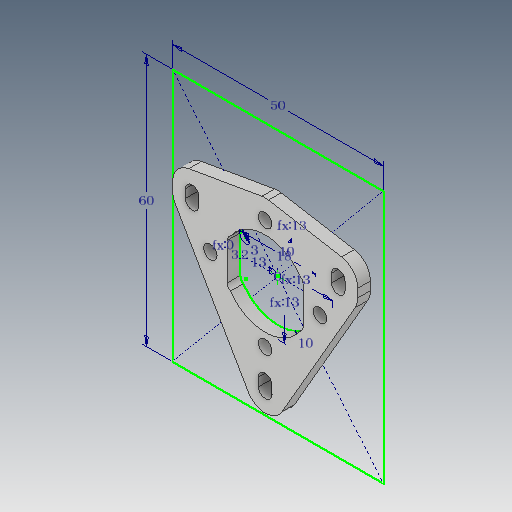
# Autodesk Inventor part: RS555-71Mount
Saved by Autodesk Inventor 2019.4 (Build 234330000, 330)
## iProperties
Created: 2019-06-16
Part Number: RS555-71Mount
Material: Generic
Document SubType Name: Modeling
Designer: AzLIer
Density: 1 g/cm^3
Appearance: Default
Mass: 2.48258 g
Surface Area: 25.0172 cm^2
Volume: 2.48258 cm^3
Author: AzLIer
Autodesk Inventor part; units mm, degrees
ref_plane "YZ Plane" through (0, 0, 0) normal (1, 0, 0) x (0, 1, 0)
ref_plane "XZ Plane" through (0, 0, 0) normal (0, 1, 0) x (-1, 0, 0)
ref_plane "XY Plane" through (0, 0, 0) normal (0, 0, 1) x (1, 0, 0)
sketch "スケッチ1" plane through (0, 0, 0) normal (0, 0, 1) x (1, 0, 0)
  line L0 (9, -4.3589) -> (9, 4.3589)
  line L1 (-9, 4.3589) -> (-9, -4.3589)
  arc A0 (8.2425, 5.6622) -> (-8.2425, 5.6622) centre (0, 0) ccw
  arc A1 (-8.2425, 5.6622) -> (-9, 4.3589) centre (-7.5, 4.3589) ccw
  arc A2 (9, 4.3589) -> (8.2425, 5.6622) centre (7.5, 4.3589) ccw
  arc A3 (8.2425, -5.6622) -> (9, -4.3589) centre (7.5, -4.3589) ccw
  arc A4 (-9, -4.3589) -> (-8.2425, -5.6622) centre (-7.5, -4.3589) ccw
  arc A5 (-8.2425, -5.6622) -> (8.2425, -5.6622) centre (0, 0) ccw
  line L2 (-9, 0) -> (9, 0) construction
  line L3 (-13, 0) -> (-13, 0) construction
  line L4 (-14.6, 0) -> (-14.6, 0)
  line L5 (-11.4, 0) -> (-11.4, 0)
  arc A6 (-11.4, 0) -> (-14.6, 0) centre (-13, 0) ccw
  arc A7 (-14.6, 0) -> (-11.4, 0) centre (-13, 0) ccw
  line L6 (25, -30) -> (-25, -30)
  line L7 (-25, -30) -> (-25, 30)
  line L8 (-25, 30) -> (25, 30)
  line L9 (25, 30) -> (25, -30)
  line L10 (25, -30) -> (-25, 30) construction
  line L11 (-25, -30) -> (25, 30) construction
  line L12 (13, 0) -> (13, 0) construction
  line L13 (11.4, 0) -> (11.4, 0)
  line L14 (14.6, 0) -> (14.6, 0)
  arc A8 (14.6, 0) -> (11.4, 0) centre (13, 0) ccw
  arc A9 (11.4, 0) -> (14.6, 0) centre (13, 0) ccw
  line L15 (0, 13) -> (0, 13) construction
  line L16 (-1.6, 13) -> (-1.6, 13)
  line L17 (1.6, 13) -> (1.6, 13)
  arc A10 (1.6, 13) -> (-1.6, 13) centre (0, 13) ccw
  arc A11 (-1.6, 13) -> (1.6, 13) centre (0, 13) ccw
  line L18 (0, -13) -> (0, -13) construction
  line L19 (1.6, -13) -> (1.6, -13)
  line L20 (-1.6, -13) -> (-1.6, -13)
  arc A12 (-1.6, -13) -> (1.6, -13) centre (0, -13) ccw
  arc A13 (1.6, -13) -> (-1.6, -13) centre (0, -13) ccw
  point P0 (0, 0)
  point P1 (0, 13)
  point P2 (0, -13)
  dimension "d2" = 18
  dimension "d3" = 3
  dimension "d5" = 10
  dimension "d6" = 0
  dimension "d7" = 10
  dimension "d8" = 3.2
  dimension "d9" = 13
  dimension "d10" = 0
  dimension "d11" = 50
  dimension "d12" = 60
  dimension "d22" = 13
  dimension "d23" = 13
  dimension "d24" = 13
  constraints: 50 end point, 31 point on circle, 20 tangent, 14 centre point, 11 midpoint, 7 parallel, 6 equal radius, 5 vertical, 4 coincident, 3 equal length, 2 horizontal, 2 horizontal alignment, 1 perpendicular, 1 point on line, 1 vertical alignment, 1 other
  measures "d2" distance between parallel lines of L0 L1
  measures "d3" diameter of A1
  measures "d5" radius of A0
  measures "d6" distance of A0.centre A5.centre
  measures "d7" radius of A5
  measures "d8" diameter of A7
  measures "d9" distance from line of A0.centre L3
  measures "d10" distance of L3.start L3.end
  measures "d11" distance of L7.end L8.end
  measures "d12" distance of L6.end L7.end
  measures "d22" distance of A0.centre L12.start
  measures "d23" distance of L15.start A0.centre
  measures "d24" distance of point (0, 0) L18.start
extrude "押し出し1" add sketch "スケッチ1" along normal blind 3
sketch "スケッチ3" plane through (0, 0, 3) normal (0, 0, 1) x (1, 0, 0)
  line L0 (0, -22) -> (0, -20) construction
  line L1 (1.6, -22) -> (1.6, -20)
  line L2 (-1.6, -20) -> (-1.6, -22)
  arc A0 (-1.6, -22) -> (1.6, -22) centre (0, -22) ccw
  arc A1 (1.6, -20) -> (-1.6, -20) centre (0, -20) ccw
  line L3 (-17.3205, 10) -> (-17.3205, 8) construction
  line L4 (-18.9205, 10) -> (-18.9205, 8)
  line L5 (-15.7205, 8) -> (-15.7205, 10)
  arc A2 (-15.7205, 10) -> (-18.9205, 10) centre (-17.3205, 10) ccw
  arc A3 (-18.9205, 8) -> (-15.7205, 8) centre (-17.3205, 8) ccw
  line L6 (17.3205, 10) -> (17.3205, 8) construction
  line L7 (15.7205, 10) -> (15.7205, 8)
  line L8 (18.9205, 8) -> (18.9205, 10)
  arc A4 (18.9205, 10) -> (15.7205, 10) centre (17.3205, 10) ccw
  arc A5 (15.7205, 8) -> (18.9205, 8) centre (17.3205, 8) ccw
  circle A6 centre (0, 0) radius 20 construction
  point P0 (0, -21)
  point P1 (-17.3205, 9)
  point P2 (17.3205, 9)
  dimension "d26" = 2
  dimension "d27" = 1.6
  dimension "d28" = 20
  dimension "d29" = 120
  constraints: 24 end point, 15 point on circle, 12 tangent, 7 centre point, 6 parallel, 3 midpoint, 2 equal radius, 2 vertical, 1 coincident, 1 vertical alignment, 1 other
  measures "d26" distance of L0.start L0.end
  measures "d27" radius of A1
  measures "d28" distance of point (0, 0) L0.end
extrude "押し出し4" cut sketch "スケッチ3" against normal blind 3
sketch "スケッチ4" plane through (0, 0, 3) normal (0, 0, 1) x (1, 0, 0)
  arc A0 (-18.9205, 8) -> (-15.7205, 8) centre (-17.3205, 8) ccw projected
  line L0 (-18.9205, 8) -> (-18.9205, 10) projected
  arc A1 (-15.7205, 10) -> (-18.9205, 10) centre (-17.3205, 10) ccw projected
  line L1 (-15.7205, 10) -> (-15.7205, 8) projected
  arc A2 (1.6, -20) -> (-1.6, -20) centre (0, -20) ccw projected
  line L2 (1.6, -20) -> (1.6, -22) projected
  arc A3 (-1.6, -22) -> (1.6, -22) centre (0, -22) ccw projected
  line L3 (-1.6, -22) -> (-1.6, -20) projected
  arc A4 (15.7205, 8) -> (18.9205, 8) centre (17.3205, 8) ccw projected
  line L4 (15.7205, 8) -> (15.7205, 10) projected
  arc A5 (18.9205, 10) -> (15.7205, 10) centre (17.3205, 10) ccw projected
  line L5 (18.9205, 10) -> (18.9205, 8) projected
  arc A6 (8.2425, -5.6622) -> (9, -4.3589) centre (7.5, -4.3589) ccw projected
  arc A7 (-8.2425, -5.6622) -> (8.2425, -5.6622) centre (0, 0) ccw projected
  arc A8 (-9, -4.3589) -> (-8.2425, -5.6622) centre (-7.5, -4.3589) ccw projected
  line L6 (-9, -4.3589) -> (-9, 4.3589) projected
  arc A9 (-8.2425, 5.6622) -> (-9, 4.3589) centre (-7.5, 4.3589) ccw projected
  arc A10 (8.2425, 5.6622) -> (-8.2425, 5.6622) centre (0, 0) ccw projected
  arc A11 (9, 4.3589) -> (8.2425, 5.6622) centre (7.5, 4.3589) ccw projected
  line L7 (9, 4.3589) -> (9, -4.3589) projected
  circle A12 centre (0, -13) radius 1.6 projected
  circle A13 centre (0, 13) radius 1.6 projected
  circle A14 centre (13, 0) radius 1.6 projected
  circle A15 centre (-13, 0) radius 1.6 projected
  line L8 (-25, -30) -> (25, -30) projected
  line L9 (25, -30) -> (25, 30) projected
  line L10 (25, 30) -> (-25, 30) projected
  line L11 (-25, 30) -> (-25, -30) projected
  arc A16 (-21.9205, 8) -> (-12.7205, 8) centre (-17.3205, 8) ccw
  line L12 (-21.9205, 8) -> (-21.9205, 10)
  arc A17 (-12.7205, 10) -> (-21.9205, 10) centre (-17.3205, 10) ccw
  line L13 (-12.7205, 10) -> (-12.7205, 8)
  line L14 (12.7205, 10) -> (12.7205, 8)
  arc A18 (12.7205, 8) -> (21.9205, 8) centre (17.3205, 8) ccw
  line L15 (21.9205, 8) -> (21.9205, 10)
  arc A19 (21.9205, 10) -> (12.7205, 10) centre (17.3205, 10) ccw
  circle A20 centre (0, 13) radius 4.6
  arc A21 (4.6, -20) -> (-4.6, -20) centre (0, -20) ccw
  line L16 (4.6, -20) -> (4.6, -22)
  arc A22 (-4.6, -22) -> (4.6, -22) centre (0, -22) ccw
  line L17 (-4.6, -22) -> (-4.6, -20)
  line L18 (-3.9837, -24.3) -> (-21.3042, 5.7)
  line L19 (3.9837, -24.3) -> (21.3042, 5.7)
  line L20 (0.7851, 17.5325) -> (18.1056, 14.5325)
  line L21 (-0.7851, 17.5325) -> (-18.1056, 14.5325)
  dimension "d32" = 3
  dimension "d33" = 3
  dimension "d34" = 3
  dimension "d35" = 3
  constraints: 20 end point, 20 point on circle, 8 tangent, 7 centre point, 9 other
  measures "d32" distance between parallel lines of L1 L13
  measures "d33" radial gap between concentric circles of A5 A19
  measures "d34" radial gap between concentric circles of A13 A20
  measures "d35" radial gap between concentric circles of A2 A21
extrude "押し出し5" cut sketch "スケッチ4" against normal blind 3 contours L0 A1 L1 A0 | L2 A3 L3 A2 | L4 A5 L5 A4 | A7 A8 L6 A9 A10 A20 A11 L7 A6 | A6 L7 A11 A10 A20 L20 A19 L14 A18 L19 A22 L16 A21 L17 L18 A16 L13 A17 L21 A9 L6 A8 A7 | A20 A10 | A10 A20 | A17 L13 A16 L12 | A19 L15 A18 L14 | A22 L17 A21 L16 | A12 | A13 | A14 | A15 keep common part
equation "\"d22\" = d9"
equation "\"d23\" = d9"
equation "\"d24\" = d23 + d10"
